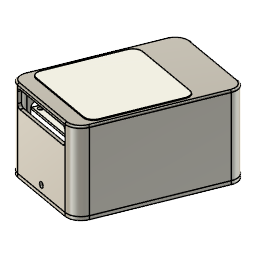
ControllerCase (Autodesk Fusion 360 design; units mm, degrees)
part number: 2026-06-22-16-49-25-115
Autodesk Fusion 360 part; units mm, degrees
sketch "スケッチ1" plane through (0, 0, 0) normal (0, 0, 1) x (1, 0, 0)
  line L0 (36, -23.5) -> (-36, -23.5)
  line L1 (-36, -23.5) -> (-36, 23.5)
  line L2 (-36, 23.5) -> (36, 23.5)
  line L3 (36, 23.5) -> (36, -23.5)
  line L4 (36, -23.5) -> (-36, 23.5) construction
  line L5 (-36, -23.5) -> (36, 23.5) construction
  line L6 (0, 0) -> (100, 0) construction
  line L7 (0, 0) -> (0, 75) construction
  line L8 (-36, 20.5) -> (-29, 20.5) construction
  line L9 (-33, 23.5) -> (-33, 16) construction
  circle A0 centre (-33, 20.5) radius 1.6
  circle A1 centre (33, 20.5) radius 1.6
  circle A2 centre (-33, -20.5) radius 1.6
  circle A3 centre (33, -20.5) radius 1.6
  line L10 (11.43, 49) -> (11.43, -29) construction
  line L11 (17.43, 45) -> (17.43, -29) construction
  line L12 (-7.57, 45) -> (-7.57, -29) construction
  line L13 (0, 0) -> (-48, 0) construction
  line L14 (19.43, -27) -> (-34.57, -27)
  line L15 (-34.57, -27) -> (-34.57, 27)
  line L16 (-34.57, 27) -> (19.43, 27)
  line L17 (19.43, 27) -> (19.43, -27)
  line L18 (19.43, -27) -> (-34.57, 27) construction
  line L19 (-34.57, -27) -> (19.43, 27) construction
  line L20 (44, -30) -> (-44, -30)
  line L21 (-44, -30) -> (-44, 30)
  line L22 (-44, 30) -> (44, 30)
  line L23 (44, 30) -> (44, -30)
  line L24 (44, -30) -> (-44, 30) construction
  line L25 (-44, -30) -> (44, 30) construction
  point P0 (-7.57, 0)
  dimension "d1" = 72
  dimension "d2" = 47
  dimension "d3" = 3
  dimension "d4" = 3
  dimension "d5" = 3.2
  dimension "d6" = 11.43
  dimension "d7" = 6
  dimension "d8" = 25
  dimension "d9" = 54
  dimension "d10" = 54
  dimension "d11" = 88
  dimension "d12" = 60
  constraint horizontal L0
  constraint perpendicular L0 L1
  constraint parallel L0 L2
  constraint parallel L1 L3
  constraint coincident L4 L6.start
  constraint coincident L5 L6.start
  constraint coincident L6.start L7.start
  constraint horizontal L6
  constraint perpendicular L6 L7
  constraint perpendicular L1 L8
  constraint perpendicular L2 L9
  constraint coincident L1 L8.start
  constraint coincident L2 L9.start
  constraint coincident L8 A0.centre
  constraint coincident L9 A0.centre
  constraint symmetric L7 A0 A1
  constraint symmetric L6 A0 A2
  constraint symmetric L6 A1 A3
  constraint perpendicular L0 L10
  constraint perpendicular L0 L11
  constraint vertical L12
  constraint parallel L6 L13
  constraint horizontal L14
  constraint perpendicular L14 L15
  constraint parallel L14 L16
  constraint parallel L15 L17
  constraint coincident L18 P0
  constraint coincident L19 P0
  constraint coincident L13 P0
  constraint coincident L12 P0
  constraint horizontal L20
  constraint perpendicular L20 L21
  constraint parallel L20 L22
  constraint parallel L21 L23
  constraint coincident L24 L6.start
  constraint coincident L25 L6.start
  measures "d1" distance of L1.end L2.end
  measures "d2" distance of L0.end L1.end
  measures "d3" distance of L2 L8
  measures "d4" distance of L1 L9
  measures "d5" diameter of A0
  measures "d6" distance of L7 L10
  measures "d7" distance of L10 L11
  measures "d8" distance of L11 L12
  measures "d9" distance of L15.end L16.end
  measures "d10" distance of L14.end L15.end
  measures "d11" distance of L21.end L22.end
  measures "d12" distance of L20.end L21.end
extrude "押し出し1" add sketch "スケッチ1" against normal blind 2 contours L0 L2 L3 L17 | L0 L14 L15 L17 | L0 L2 A0 A2 L15 L17 | L0 L1 L2 A0 A2 L15 | L2 L15 L16 L17 | L20 L21 L22 L23 makes body 1
fillet "フィレット1" radius 8 4 edges at (-44, -30, -1) (44, -30, -1) (44, 30, -1) (-44, 30, -1) on bodies 1
sketch "スケッチ3" plane through (0, 0, -2) normal (0, 0, -1) x (1, 0, 0)
  arc A0 (-44, -22) -> (-36, -30) centre (-36, -22) ccw
  line L0 (-36, -30) -> (36, -30)
  arc A1 (36, -30) -> (44, -22) centre (36, -22) ccw
  line L1 (44, -22) -> (44, 22)
  arc A2 (44, 22) -> (36, 30) centre (36, 22) ccw
  line L2 (36, 30) -> (-36, 30)
  arc A3 (-36, 30) -> (-44, 22) centre (-36, 22) ccw
  line L3 (-44, 22) -> (-44, -22)
  circle A4 centre (33, -20.5) radius 1.6
  circle A5 centre (-33, -20.5) radius 1.6
  circle A6 centre (-33, 20.5) radius 1.6
  circle A7 centre (33, 20.5) radius 1.6
  line L4 (0, 0) -> (0, -35) construction
  line L5 (0, 0) -> (-50, 0) construction
  circle A8 centre (33, -20.5) radius 5
  circle A9 centre (33, -20.5) radius 3
  circle A10 centre (-33, -20.5) radius 3
  circle A11 centre (-33, -20.5) radius 5
  circle A12 centre (33, 20.5) radius 5
  circle A13 centre (33, 20.5) radius 3
  circle A14 centre (-33, 20.5) radius 5
  circle A15 centre (-33, 20.5) radius 3
  dimension "d19" = 10
  dimension "d20" = 6
  constraint coincident L4.start L5.start
  constraint vertical L4
  constraint perpendicular L4 L5
  constraint concentric A4 A8
  constraint concentric A8 A9
  constraint symmetric L4 A8 A11
  constraint symmetric L4 A9 A10
  constraint symmetric L5 A8 A12
  constraint symmetric L5 A9 A13
  constraint symmetric L5 A10 A15
  constraint symmetric L5 A11 A14
  measures "d19" diameter of A8
  measures "d20" diameter of A9
extrude "押し出し2" add sketch "スケッチ3" against normal blind 5 contours A8 | A9 | A10 | A11 | A12 | A13 | A14 | A15 bodies 1
extrude "押し出し3" cut sketch "スケッチ3" against normal blind 3 contours A9 | A10 | A13 | A15 bodies 1
extrude "押し出し4" add sketch "スケッチ1" along normal blind 1.2 separate body contours L0 L2 L3 L17 | L0 L2 A0 A2 L15 L17 | L0 L1 L2 A0 A2 L15 makes body 2
move_body "移動1" bodies 2 to x (1, 0, 0) y (0, 1, 0) z (0, 0, 1) at (0, 0, 8)
copy_body "ボディのコピーと貼り付け1" bodies 2 makes body 3
move_body "移動2" bodies 3 to x (1, 0, 0) y (0, 1, 0) z (0, 0, 1) at (0, 0, 21.2)
extrude "押し出し5" add sketch "スケッチ1" along normal blind 12.6 separate body contours L0 L14 L15 L17 | L0 L2 A0 A2 L15 L17 | L2 L15 L16 L17 | A2 L15 | A0 L15 picked at (-32.4709, -20.9956) picked at (-33.7418, 21.0229) makes body 4
move_body "移動3" bodies 4 to x (1, 0, 0) y (0, 1, 0) z (0, 0, 1) at (0, 0, 32.8)
fillet "フィレット2" radius 5 4 edges at (19.43, -27, 39.1) (19.43, 27, 39.1) (-34.57, -27, 39.1) (-34.57, 27, 39.1) on bodies 4
extrude "押し出し6" add sketch "スケッチ1" along normal blind 45 separate body contours L0 L2 L3 L17 | L0 L14 L15 L17 | L0 L2 A0 A2 L15 L17 | L0 L1 L2 A0 A2 L15 | L2 L15 L16 L17 | A2 L15 | A2 L15 | A0 L15 | A0 L15 | A1 | A3 | L20 L21 L22 L23 makes body 5
fillet "フィレット3" radius 8 4 edges at (-44, -30, 22.5) (44, -30, 22.5) (44, 30, 22.5) (-44, 30, 22.5) on bodies 5
fillet "フィレット7" radius 1 8 edges at (-41.6569, -27.6569, 45) (0, -30, 45) (41.6569, -27.6569, 45) (44, 0, 45) (41.6569, 27.6569, 45) (0, 30, 45) (-41.6569, 27.6569, 45) (-44, 0, 45) on bodies 5
shell "シェル1" thickness 2 removed faces 1 at (12, -10, 0) on bodies 5
combine "結合1" operation cut target body 5 tool bodies 4 keep tools
sketch "スケッチ4" plane through (0, 30, 0) normal (0, 1, 0) x (-1, 0, 0)
  line L0 (36, 0) -> (36, 44)
  line L1 (-36, 44) -> (-36, 0)
  line L2 (-36, 0) -> (36, 0)
  line L3 (0, 0) -> (0, 50) construction
  line L4 (0, 8) -> (-34, 8)
  line L5 (-34, 8) -> (-34, 30.4)
  line L6 (-34, 30.4) -> (0, 30.4)
  line L7 (0, 30.4) -> (0, 8)
  line L8 (0, 0) -> (-50, 0) construction
  line L9 (34, 30.4) -> (0, 30.4)
  line L10 (34, 8) -> (34, 30.4)
  line L11 (0, 8) -> (34, 8)
  line L12 (-36, 8) -> (36, 8)
  line L13 (36, 8) -> (36, 9.2)
  line L14 (36, 9.2) -> (-36, 9.2)
  line L15 (-36, 9.2) -> (-36, 8)
  line L16 (-36, 29.2) -> (36, 29.2)
  line L17 (36, 29.2) -> (36, 30.4)
  line L18 (36, 30.4) -> (-36, 30.4)
  line L19 (-36, 30.4) -> (-36, 29.2)
  line L20 (-19.43, 45.4) -> (-14.43, 45.4)
  line L21 (-19.43, 45.4) -> (-19.43, 32.8)
  line L22 (-14.43, 32.8) -> (-19.43, 32.8)
  line L23 (-14.43, 32.8) -> (-14.43, 45.4)
  line L24 (29.57, 32.8) -> (29.57, 45.4)
  line L25 (29.57, 45.4) -> (-14.43, 45.4)
  line L26 (-14.43, 45.4) -> (-14.43, 32.8)
  line L27 (-14.43, 32.8) -> (29.57, 32.8)
  line L28 (29.57, 45.4) -> (34.57, 45.4)
  line L29 (29.57, 45.4) -> (29.57, 32.8)
  line L30 (34.57, 32.8) -> (29.57, 32.8)
  line L31 (34.57, 32.8) -> (34.57, 45.4)
  line L32 (36, 44) -> (-36, 44)
  line L33 (-34, 8) -> (-34, 0)
  line L34 (34, 8) -> (34, 0)
  dimension "d36" = 34
  dimension "d37" = 8
  dimension "d38" = 22.4
  dimension "d41" = 20
  dimension "d42" = 2.4
  constraint coincident L3.start L8.start
  constraint horizontal L4
  constraint vertical L5
  constraint horizontal L6
  constraint vertical L7
  constraint coincident L3 L4.start
  constraint perpendicular L3 L8
  constraint symmetric L3 L4.start L7.end
  constraint symmetric L3 L4.end L10.start
  constraint symmetric L3 L5.end L9.start
  constraint symmetric L3 L6.end L7.start
  constraint coincident L8 L33.end
  constraint coincident L2 L34.end
  constraint perpendicular L2 L34
  constraint perpendicular L8 L33
  measures "d36" distance of L4.start L4.end
  measures "d37" distance of L4 L8
  measures "d38" distance of L4 L6
  measures "d41" distance of L14 L16
  measures "d42" distance of L18 L27
extrude "押し出し7" cut sketch "スケッチ4" against normal blind 2 contours L2 L4 L11 L12 L33 L34 | L7 L10 L11 L12 L14 | L7 L10 L14 L16 | L4 L5 L7 L12 L14 | L7 L9 L10 L16 L18 | L5 L7 L14 L16 | L5 L6 L7 L16 L18 bodies 5
fillet "フィレット4" radius 3 2 edges at (34, 29, 30.4) (-34, 29, 30.4) on bodies 5
sketch "スケッチ5" plane through (-44, 0, 0) normal (-1, 0, 0) x (0, -1, 0)
  line L0 (-22, 44) -> (-22, 0)
  line L1 (-22, 0) -> (22, 0)
  line L2 (22, 0) -> (22, 44)
  line L3 (-27, 45.4) -> (-22, 45.4)
  line L4 (-27, 45.4) -> (-27, 32.8)
  line L5 (-22, 32.8) -> (-27, 32.8)
  line L6 (-22, 32.8) -> (-22, 45.4)
  line L7 (-22, 45.4) -> (-22, 32.8)
  line L8 (-22, 32.8) -> (22, 32.8)
  line L9 (22, 32.8) -> (22, 45.4)
  line L10 (22, 45.4) -> (-22, 45.4)
  line L11 (22, 45.4) -> (27, 45.4)
  line L12 (22, 45.4) -> (22, 32.8)
  line L13 (27, 32.8) -> (22, 32.8)
  line L14 (27, 32.8) -> (27, 45.4)
  line L15 (-30, 44) -> (-30, 0)
  line L16 (-22, 0) -> (-30, 0)
  line L17 (-22, 0) -> (-22, 44)
  line L18 (22, 44) -> (22, 0)
  line L19 (30, 0) -> (22, 0)
  line L20 (30, 0) -> (30, 44)
  line L21 (-22, 32.8) -> (22, 32.8)
  line L22 (22, 32.8) -> (22, 42.8)
  line L23 (22, 42.8) -> (-22, 42.8)
  line L24 (-22, 42.8) -> (-22, 32.8)
  line L25 (22, 44) -> (-22, 44)
  line L26 (-22, 44) -> (-30, 44)
  line L27 (30, 44) -> (22, 44)
  dimension "d45" = 10
  dimension "d46" = 44
  constraint horizontal L21
  constraint vertical L22
  constraint horizontal L23
  constraint vertical L24
  constraint coincident L5.start L6.start
  measures "d45" distance of L5.start L23.end
  measures "d46" distance of L22 L24
extrude "押し出し8" cut sketch "スケッチ5" against normal blind 5 contours L0 L2 L6 L7 L8 L9 L12 L17 L18 L21 L22 L23 L24 bodies 5
fillet "フィレット5" radius 2 4 edges at (-43, 22, 32.8) (-43, -22, 32.8) (-43, 22, 42.8) (-43, -22, 42.8) on bodies 5
sketch "スケッチ6" plane through (0, 0, 0) normal (0, 0, 1) x (1, 0, 0)
  circle A0 centre (-33, 20.5) radius 5
  circle A1 centre (33, -20.5) radius 5
  circle A2 centre (-33, -20.5) radius 5
  circle A3 centre (33, 20.5) radius 5
  arc A4 (-36, 30) -> (-44, 22) centre (-36, 22) ccw
  line L0 (-44, 22) -> (-44, -22)
  arc A5 (-44, -22) -> (-36, -30) centre (-36, -22) ccw
  line L1 (-36, -30) -> (36, -30)
  arc A6 (36, -30) -> (44, -22) centre (36, -22) ccw
  line L2 (44, -22) -> (44, 22)
  arc A7 (44, 22) -> (36, 30) centre (36, 22) ccw
  line L3 (36, 30) -> (-36, 30)
  circle A8 centre (-33, -20.5) radius 1.6
  circle A9 centre (33, -20.5) radius 1.6
  circle A10 centre (33, 20.5) radius 1.6
  circle A11 centre (-33, 20.5) radius 1.6
  line L4 (36, 23.5) -> (-36, 23.5)
  line L5 (-36, 23.5) -> (-36, -23.5)
  line L6 (-36, -23.5) -> (36, -23.5)
  line L7 (36, -23.5) -> (36, 23.5)
  line L8 (-42, 22) -> (-42, -22)
  line L9 (0, 0) -> (-50, 0) construction
  line L10 (-42, 0) -> (-37, 0)
  line L11 (-37, 0) -> (-37, 15)
  line L12 (-37, 15) -> (-42, 15)
  line L13 (-42, 15) -> (-42, 0)
  line L14 (-42, -15) -> (-42, 0)
  line L15 (-37, -15) -> (-42, -15)
  line L16 (-37, 0) -> (-37, -15)
  line L17 (0, 0) -> (0, 30) construction
  line L18 (37, 15) -> (42, 15)
  line L19 (42, 22) -> (42, -22)
  line L20 (37, -15) -> (42, -15)
  line L21 (37, 0) -> (37, -15)
  line L22 (37, 0) -> (37, 15)
  dimension "d51" = 8
  dimension "d52" = 2
  dimension "d55" = 15
  dimension "d56" = 5
  constraint vertical L8
  constraint coincident L9.start L17.start
  constraint horizontal L9
  constraint horizontal L10
  constraint vertical L11
  constraint horizontal L12
  constraint vertical L13
  constraint midpoint L8 L10.start
  constraint symmetric L9 L10.start L13.end
  constraint symmetric L9 L10.end L11.start
  constraint symmetric L9 L11.end L15.start
  constraint symmetric L9 L12.end L14.start
  constraint collinear L9 L10
  constraint midpoint L3 L17.end
  constraint symmetric L8.start L17 L19.start
  constraint symmetric L8.end L17 L19.end
  constraint symmetric L10.end L17 L21.start
  constraint symmetric L11.end L17 L18.start
  constraint symmetric L12.end L17 L18.end
  constraint symmetric L14.start L17 L20.end
  constraint symmetric L15.start L17 L20.start
  measures "d51" distance of L0 L5
  measures "d52" distance of L0 L8
  measures "d55" distance of L10.start L12.end
  measures "d56" distance of L11 L13
extrude "押し出し9" add sketch "スケッチ6" along normal blind 8 contours L8 L10 L11 L12 L13 | L8 L10 L14 L15 L16 | L18 L19 L20 L21 L22 bodies 1
extrude "押し出し10" cut 1 faces at (-42, 5, 2.6667) along direction (1, 0, 0) blind 0.15 on bodies 1 bodies 1
extrude "押し出し11" cut 1 faces at (42, 5, 2.6667) along direction (-1, 0, 0) blind 0.15 on bodies 1 bodies 1
fillet "フィレット6" radius 1 8 edges at (-39.425, -15, 0) (-39.425, -15, 8) (-39.425, 15, 8) (-39.425, 15, 0) (39.425, 15, 0) (39.425, 15, 8) (39.425, -15, 8) (39.425, -15, 0) on bodies 1
sketch "スケッチ7" plane through (-44, 0, 0) normal (-1, 0, 0) x (0, -1, 0)
  line L0 (20, 32.8) -> (-20, 32.8)
  arc A0 (-22, 34.8) -> (-20, 32.8) centre (-20, 34.8) ccw
  line L1 (-22, 34.8) -> (-22, 0)
  line L2 (-22, 0) -> (22, 0)
  line L3 (22, 0) -> (22, 34.8)
  arc A1 (20, 32.8) -> (22, 34.8) centre (20, 34.8) ccw
  arc A2 (-14, 8) -> (-15, 7) centre (-14, 7) ccw
  line L4 (-15, 7) -> (-15, 1)
  arc A3 (-16, 0) -> (-15, 1) centre (-16, 1) ccw
  line L5 (-16, 0) -> (16, 0)
  arc A4 (15, 1) -> (16, 0) centre (16, 1) ccw
  line L6 (15, 1) -> (15, 7)
  arc A5 (15, 7) -> (14, 8) centre (14, 7) ccw
  line L7 (14, 8) -> (-14, 8)
  line L8 (0, 0) -> (0, 15) construction
  line L9 (-15, 4) -> (15, 4) construction
  circle A6 centre (0, 4) radius 1.6
  circle A7 centre (0, 4) radius 1.25
  dimension "d65" = 8
  dimension "d66" = 4
  dimension "d67" = 3.2
  dimension "d68" = 2.5
  constraint coincident L8.start origin
  constraint perpendicular L2 L8
  constraint midpoint L4 L9.start
  constraint midpoint L6 L9.end
  constraint midpoint L9 A6.centre
  constraint concentric A6 A7
  measures "d65" distance of L5 L7
  measures "d66" distance of L5 L9
  measures "d67" diameter of A6
  measures "d68" diameter of A7
extrude "押し出し12" cut sketch "スケッチ7" against normal blind 117 contours A6 | A7 bodies 5
extrude "押し出し13" cut sketch "スケッチ7" against normal blind 98 contours A7 bodies 1
fillet "フィレット8" radius 1 8 edges at (40.2426, -26.2426, 43) (42, 0, 43) (40.2426, 26.2426, 43) (0, 28, 43) (-40.2426, 26.2426, 43) (-42, 0, 43) (-40.2426, -26.2426, 43) (0, -28, 43) on bodies 5
move_face "面をオフセット1" offset -0.15 8 faces at (-14.9033, 27, 44.3333) (-34.4271, 23.1868, 44.3333) (-34.57, 7.3333, 43.6667) (19.43, 7.3333, 44.3333) (-14.9033, -27, 44.3333) (-30.5169, -26.9095, 43.6667) (15.3769, 26.9095, 44.3333) (15.6168, -26.8571, 44.3333) on bodies 5
named bodies: "bottom", "仮_基板1", "仮_基板2", "仮_M5Stack", "top"
